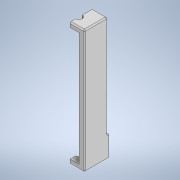
# Autodesk Inventor part: lead_screw_housing
Saved by Autodesk Inventor 2021 (Build 250183000, 183)
## iProperties
Created: 2021-03-03
Part Number: lead_screw_housing
Material: Generic
Document SubType Name: Modeling
Designer: dsdan
Density: 1 g/cm^3
Appearance: Default
Author: dsdan
Autodesk Inventor part; units mm, degrees
ref_plane "YZ Plane" through (0, 0, 0) normal (1, 0, 0) x (0, 1, 0)
ref_plane "XZ Plane" through (0, 0, 0) normal (0, 1, 0) x (-1, 0, 0)
sketch "Sketch1" plane through (0, 0, 0) normal (0, 1, 0) x (-1, 0, 0)
  line L0 (0, 0) -> (-7.5, 0)
  line L1 (-7.5, -15) -> (0, -15)
  line L2 (0, -15) -> (0, 0)
  line L3 (-7.5, -9.5) -> (-9.5, -9.5)
  line L4 (-9.5, -9.5) -> (-9.5, -5.5)
  line L5 (-9.5, -5.5) -> (-7.5, -5.5)
  line L6 (-7.5, 0) -> (-7.5, -5.5)
  line L7 (-7.5, -9.5) -> (-7.5, -15)
  line L8 (-7.6, -15.1) -> (0.1, -15.1)
  line L9 (0.1, -15.1) -> (0.1, 0.1)
  line L10 (0.1, 0.1) -> (-7.6, 0.1)
  line L11 (-7.6, 0.1) -> (-7.6, -5.4)
  line L12 (-7.6, -5.4) -> (-9.6, -5.4)
  line L13 (-9.6, -5.4) -> (-9.6, -9.6)
  line L14 (-9.6, -9.6) -> (-7.6, -9.6)
  line L15 (-7.6, -9.6) -> (-7.6, -15.1)
  line L16 (0, 0) -> (-12.1, 0)
  line L17 (-12.1, 0) -> (-12.1, -19.6)
  line L18 (-12.1, -19.6) -> (0, -19.6)
  line L19 (0, -19.6) -> (0, 0)
  point P0 (-7.6, 0)
  point P1 (0, -15.1)
  dimension "d2" = 7.5
  dimension "d3" = 15
  dimension "d8" = 4
  dimension "d9" = 2
  dimension "d10" = 5.5
  dimension "d11" = 0.1
  dimension "d12" = 4.5
  dimension "d13" = 4.5
  constraints: 40 end point, 10 parallel, 7 perpendicular, 3 horizontal, 2 collinear, 7 other
  measures "d2" distance of L1.start L1.end
  measures "d3" distance of L0.end L1.start
  measures "d8" distance of L3.end L4.end
  measures "d9" distance of L3.start L3.end
  measures "d10" distance of L3.start L1.start
  measures "d11" distance between parallel lines of L7 L15
  measures "d12" distance between parallel lines of L11 L17
  measures "d13" distance between parallel lines of L8 L18
extrude "Extrusion1" add sketch "Sketch1" along normal blind 96.1 contours L11 L12 L13 L14 L15 L8 L19 L18 L17 L16
ref_plane "Work Plane1" through (0, 48.05, 0) normal (0, -1, 0) x (1, 0, 0)
sketch "Sketch2" plane through (0, 96.1, 0) normal (0, 1, 0) x (1, 0, 0)
  line L0 (7.6, 9.6) -> (9.6, 9.6) projected
  line L1 (9.6, 9.6) -> (9.6, 5.4) projected
  line L2 (9.6, 5.4) -> (7.6, 5.4) projected
  line L3 (7.6, 5.4) -> (7.6, 0) projected
  line L4 (7.6, 0) -> (12.1, 0) projected
  line L5 (12.1, 0) -> (12.1, 19.6) projected
  line L6 (12.1, 19.6) -> (0, 19.6) projected
  line L7 (0, 19.6) -> (0, 15.1) projected
  line L8 (0, 15.1) -> (7.6, 15.1) projected
  line L9 (7.6, 15.1) -> (7.6, 9.6) projected
  line L10 (12.1, 0) -> (12.1, 19.6) projected
  line L11 (12.1, 19.6) -> (0, 19.6)
  line L12 (0, 19.6) -> (0, 0)
  line L13 (0, 0) -> (12.1, 0)
  line L14 (12.1, 0) -> (12.1, 19.6)
  circle A0 centre (0, 7.5) radius 2.75
  line L15 (0, 7.5) -> (9.6, 7.5)
  line L16 (9.6, 9.6) -> (9.6, 5.4) projected
  point P0 (0, 10.25)
  point P1 (0, 4.75)
  dimension "d16" = 5.5
  constraints: 10 end point, 2 parallel, 2 perpendicular, 1 centre point, 1 horizontal, 1 midpoint, 1 point on line
  measures "d16" diameter of A0
extrude "Extrusion2" add sketch "Sketch2" along normal blind 3.9 contours L9 L8 L7 L6 L5 L4 L3 L2 L1 L0 | L0 L1 L15 A0 L12 L8 L9 | L1 L2 L3 L13 L12 A0 L15
mirror "Mirror1" about plane through (0, 48.05, 0) normal (0, -1, 0) of "Extrusion2"
chamfer "Chamfer1" distance 1 angle 45 2 edges at (2.75, 96.1, -7.5) (2.75, -3.9, -7.5)
sketch "Sketch5" plane through (12.1, 100, -19.6) normal (0, 0, -1) x (-1, 0, 0)
  circle A0 centre (12.1, -95.4279) radius 3.275
  line L0 (12.1, -88.9558) -> (17.705, -92.1919)
  line L1 (17.705, -92.1919) -> (17.705, -98.664)
  line L2 (17.705, -98.664) -> (12.1, -101.9)
  line L3 (12.1, -101.9) -> (6.495, -98.664)
  line L4 (6.495, -98.664) -> (6.495, -92.1919)
  line L5 (6.495, -92.1919) -> (12.1, -88.9558)
  line L6 (6.495, -92.1919) -> (17.705, -98.664) construction
  line L7 (17.705, -92.1919) -> (6.495, -98.664) construction
  line L8 (12.1, -103.9) -> (12.1, 0) projected
  dimension "d26" = 6.55
  dimension "d27" = 11.21
  dimension "d48" = 2
  constraints: 16 end point, 2 coincident, 2 point on line, 1 centre point, 13 other
  measures "d26" diameter of A0
  measures "d27" distance between parallel lines of L1 L4
  measures "d48" distance of L8.start L2.end
extrude "Extrusion3" cut sketch "Sketch5" against normal blind 2
extrude "Extrusion7" cut sketch "Sketch5" against normal through all contours A0 L8 | L8 A0
sketch "Sketch7" plane through (12.1, 100, -19.6) normal (0, 0, -1) x (-1, 0, 0)
  line L0 (0, -103.9) -> (0, 0) projected
  line L1 (12.1, -86.9558) -> (0, -86.9558)
  line L2 (0, -86.9558) -> (0, -103.9)
  line L3 (0, -103.9) -> (12.1, -103.9)
  line L4 (12.1, -103.9) -> (12.1, -86.9558)
  arc A0 (12.1, -92.1529) -> (12.1, -98.7029) centre (12.1, -95.4279) ccw projected
  line L5 (12.1, -88.9558) -> (12.1, -92.1529) projected
  line L6 (6.495, -92.1919) -> (12.1, -88.9558) projected
  line L7 (6.495, -98.664) -> (6.495, -92.1919) projected
  line L8 (12.1, -101.9) -> (6.495, -98.664) projected
  line L9 (12.1, -98.7029) -> (12.1, -101.9) projected
  line L10 (12.1, -88.9558) -> (12.1, 0) projected
  point P0 (12.1, -100)
  point P1 (12.1, -88.9558)
  point P2 (0, -86.9558)
  dimension "d51" = 2
  constraints: 8 end point, 2 parallel, 1 collinear, 1 horizontal, 1 perpendicular
  measures "d51" distance of L1.start L10.start
extrude "Extrusion8" add sketch "Sketch7" along normal blind 2 contours L0 L1 L4 L6 L7 L8 L3
chamfer "Chamfer4" distance 2 angle 45 1 edges at (6.05, 13.0442, -19.6)
chamfer "Chamfer3" distance 1 angle 45 10 edges at (6.05, -3.9, 0) (12.1, 100, -9.8) (6.05, 100, -19.6) (6.05, 100, 0) (12.1, 48.05, 0) (12.1, -3.9, -10.8) (6.05, -3.9, -21.6) (12.1, 14.0441, -20.5999) (12.1, 57.522, -19.6) (12.1, 4.5721, -21.6)
body "Solid1"
